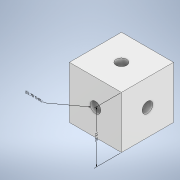
# Autodesk Inventor part: C-M3-M
Saved by Autodesk Inventor 2022 (Build 260153000, 153)
## iProperties
Company: El Camino College
Created: 2023-04-04
Part Number: C-M3-M
Material: ABS Plastic
Document SubType Name: Modeling
Designer: Edgar Tejada
Density: 1.06 g/cm^3
Appearance: Smooth - White
Mass: 2.22714 g
Surface Area: 12.8513 cm^2
Volume: 2.10107 cm^3
Author: Edgar Tejada
Title: Corner M3 Mount
Subject: Ergonomic Fight Stick
Autodesk Inventor part; units mm, degrees
ref_plane "YZ Plane" through (0, 0, 0) normal (1, 0, 0) x (0, 1, 0)
ref_plane "XZ Plane" through (0, 0, 0) normal (0, 1, 0) x (-1, 0, 0)
ref_plane "XY Plane" through (0, 0, 0) normal (0, 0, 1) x (1, 0, 0)
sketch "Sketch1" plane through (0, 0, 0) normal (0, 1, 0) x (-1, 0, 0)
  line L0 (6.6, 6.6) -> (-6.6, 6.6)
  line L1 (-6.6, 6.6) -> (-6.6, -6.6)
  line L2 (-6.6, -6.6) -> (6.6, -6.6)
  line L3 (6.6, -6.6) -> (6.6, 6.6)
  line L4 (6.6, 6.6) -> (-6.6, -6.6) construction
  line L5 (-6.6, 6.6) -> (6.6, -6.6) construction
  point P0 (0, 0)
  dimension "d0" = 13.2
  constraints: 12 end point, 2 midpoint, 2 parallel, 2 perpendicular, 1 horizontal
  measures "d0" distance of L0.start L0.end
extrude "Extrusion1" add sketch "Sketch1" along normal mid plane 13.2
sketch "Sketch2" plane through (0, 6.6, 0) normal (0, 1, 0) x (1, 0, 0)
  circle A0 centre (0, 0) radius 1.35
  dimension "d3" = 2.7
  constraints: 1 centre point, 1 coincident
  measures "d3" diameter of A0
sketch "Sketch3" plane through (6.6, -6.6, -6.6) normal (1, 0, 0) x (0, 0, -1)
  circle A0 centre (-6.6, 6.6) radius 1.35
  dimension "d4" = 2.7
  constraints: 1 centre point, 1 coincident
  measures "d4" diameter of A0
sketch "Sketch4" plane through (-6.6, 6.6, 6.6) normal (0, 0, 1) x (1, 0, 0)
  circle A0 centre (6.6, -6.6) radius 1.35
  dimension "d5" = 2.7
  constraints: 1 centre point, 1 coincident
  measures "d5" diameter of A0
extrude "Extrusion2" cut sketch "Sketch4" along normal through all both and the other way through all
extrude "Extrusion3" cut sketch "Sketch2" along normal through all both and the other way through all
extrude "Extrusion4" cut sketch "Sketch3" against normal through all
equation "\"d1\" = d0"
equation "\"d4\" = d3"
equation "\"d5\" = d3"
body "Solid1"
